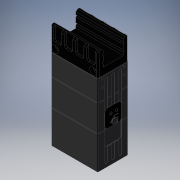
# Autodesk Inventor part: SCHUNK-5521120 Gehaeuse EGP 40
Saved by Autodesk Inventor 2019 (Build 230136000, 136)
## iProperties
Created: 2022-08-29
Part Number: SCHUNK-5521120 Gehaeuse EGP 40
Material: Generic
Catalog Web Link: www.cadenas.de
Description: EGP-Electrical 2-finger parallel gripper
Vendor: SCHUNK
Document SubType Name: Modeling
Designer: psAdmin
Manufacturer: SCHUNK
Mass: 78.9244 g
Surface Area: 169.69 cm^2
Volume: 78.9244 cm^3
Density: 1 g/cm^3
Appearance: PSOLRGB-175-175-175
Category: PARTsolutions
Company: SCHUNK
Title: SCHUNK-5521120 Gehaeuse EGP 40
Author: Cadenas PARTsolutions
Comments: Electrical 2-finger parallel gripper
PSOL_IDENT_0: {$CADENAS_DATA/23d-libs/schunk/greifsysteme/greifmodule/greifmodule_elektrisch/2_finger_parallelgrei
PSOL_IDENT_1: fer/kleinteilegreifer/egp/egp_geh.prj},197 {VTYP=3D},{NB=SCHUNK-5521120 Gehaeuse EGP 40},{LINA=SCHUN
PSOL_IDENT_2: K-5521120 Gehaeuse EGP 40},{NN=EGP},{DATE=27.06.2022 11:10:53},{GEOMDATE=27.06.2022 11:07:50},{VERSI
PSOL_IDENT_3: ON=},{LINEID=10},{WBVAR=},{WBNUMERIC=}  {NB=SCHUNK-5521120 Gehaeuse EGP 40},{LINA=SCHUNK-5521120 Geh
PSOL_IDENT_4: aeuse EGP 40},{KT=DUMMY},{IDNR=5521120},{TYP=EGP 40},{TYP1=2.000},{TYP2=2.000},{TYP3=3.000},{HUB=16.
PSOL_IDENT_5: 000},{HOEHEFIN=100.650},{LGES=40.000},{LIOL=0.000},{WIOL=0.000},{BGES=26.000},{HGES=88.400},{F1=1.00
PSOL_IDENT_6: 0},{HADG=19.750},{HGGE=18.000},{HMGE=22.600},{HDEC=28.000},{F2=0.300},{H1=13.450},{H2=9.450},{H3=6.0
PSOL_IDENT_7: 00},{B1=17.000},{B2=19.700},{T1=0.900},{F3=1.500},{L1=32.000},{H4=3.750},{D2=6.000},{T2=2.900},{D3=4
PSOL_IDENT_8: .000},{T3=6.000},{L2=10.750},{L3=7.000},{L4=2.500},{H5=11.000},{R1=1.500},{T4=1.750},{B3=18.400},{H7=
PSOL_IDENT_9: 10.000},{H8=6.000},{D7=2.500},{T7=2.500},{T8=3.900},{L6=32.000},{D9=6.000},{T9=2.900},{D10=4.000},{T
PSOL_IDENT_10: 10=8.500},{T11=10.500},{L7=34.400},{AL7=0.000},{L8=20.000},{D12=5.000},{T12=14.400},{D13=4.500},{T13=
PSOL_IDENT_11: 2.500},{SW1=2.000},{TSW1=1.100},{L10=61.100},{T14=0.300},{L11=25.000},{L12=14.600},{L13=4.250},{B4=2
PSOL_IDENT_12: .500},{B5=3.500},{D15=12.000},{L15=6.600},{B15=14.200},{B16=7.100},{B17=0.000},{H15=12.800},{R15=2.5
PSOL_IDENT_13: 00},{F4=0.100},{T15=0.600},{H16=15.400},{H17=3.400},{B18=0.650},{D16=4.600},{T16=0.800},{H18=9.900},
PSOL_IDENT_14: {B19=2.000},{B20=3.000},{D17=2.300},{LTYP=34.500},{BTYP=24.300},{TTYP=0.100},{HTYP=9.300},{ETYP=3.00
PSOL_IDENT_15: 0},{G1=3.000},{G1T=4.000},{G1K=6.000},{G1L1=15.250},{G1L2=10.000},{G2L1=0.000},{D18=0.000},{LADG=0.0
PSOL_IDENT_16: 00},{L20=0.010}
NB: SCHUNK-5521120 Gehaeuse EGP 40
NN: EGP
NT: Electrical 2-finger parallel gripper
NBSYN: SCHUNK-$IDNR. Gehaeuse $TYP.
LINA: SCHUNK-5521120 Gehaeuse EGP 40
CATALOG: SCHUNK
IDNR: 5521120
TYP: EGP 40
TYP1: 2
TYP2: 2
TYP3: 3
HUB: 16
HOEHEFIN: 100.65
LGES: 40
LIOL: 0
WIOL: 0
BGES: 26
HGES: 88.4
F1: 1
HADG: 19.75
HGGE: 18
HMGE: 22.6
HDEC: 28
F2: 0.3
H1: 13.45
H2: 9.45
H3: 6
B1: 17
B2: 19.7
T1: 0.9
F3: 1.5
L1: 32
H4: 3.75
D2: 6
T2: 2.9
D3: 4
T3: 6
L2: 10.75
L3: 7
L4: 2.5
H5: 11
R1: 1.5
T4: 1.75
B3: 18.4
H7: 10
H8: 6
D7: 2.5
T7: 2.5
T8: 3.9
L6: 32
D9: 6
T9: 2.9
D10: 4
T10: 8.5
T11: 10.5
L7: 34.4
AL7: 0
L8: 20
D12: 5
T12: 14.4
D13: 4.5
T13: 2.5
SW1: 2
TSW1: 1.1
L10: 61.1
T14: 0.3
L11: 25
L12: 14.6
L13: 4.25
B4: 2.5
B5: 3.5
D15: 12
L15: 6.6
B15: 14.2
B16: 7.1
B17: 0
H15: 12.8
R15: 2.5
F4: 0.1
T15: 0.6
H16: 15.4
H17: 3.4
B18: 0.65
D16: 4.6
T16: 0.8
H18: 9.9
B19: 2
B20: 3
D17: 2.3
LTYP: 34.5
BTYP: 24.3
TTYP: 0.1
HTYP: 9.3
ETYP: 3
G1: 3
G1T: 4
G1K: 6
G1L1: 15.25
G1L2: 10
G2L1: 0
D18: 0
LADG: 0
L20: 0.01
SUPPLIER: SCHUNK
ARTICLENO: SCHUNK-5521120 Gehaeuse EGP 40
BOMINFO: SCHUNK-5521120 Gehaeuse EGP 40
CREATOR: CADENAS GmbH
Autodesk Inventor part; units mm, degrees
sketch "Sketch_1" plane through (0, 0, 0) normal (0, 1, 0) x (-1, 0, 0)
  line L0 (20, -12) -> (20, 12)
  line L1 (20, 12) -> (19, 13)
  line L2 (19, 13) -> (-19, 13)
  line L3 (-19, 13) -> (-20, 12)
  line L4 (-20, 12) -> (-20, -12)
  line L5 (-20, -12) -> (-19, -13)
  line L6 (-19, -13) -> (19, -13)
  line L7 (19, -13) -> (20, -12)
  constraints: 16 end point
extrude "Extrusion1" add sketch "Sketch_1" along normal blind 88.4
sketch "Sketch_25" plane through (0, 88.4, 0) normal (0, 1, 0) x (1, 0, 0)
  circle A0 centre (0, 0) radius 40
  line L0 (-20, 11.9) -> (-20, -11.9)
  line L1 (-20, -11.9) -> (-18.9, -13)
  line L2 (-18.9, -13) -> (18.9, -13)
  line L3 (18.9, -13) -> (20, -11.9)
  line L4 (20, -11.9) -> (20, 11.9)
  line L5 (20, 11.9) -> (18.9, 13)
  line L6 (18.9, 13) -> (-18.9, 13)
  line L7 (-18.9, 13) -> (-20, 11.9)
  constraints: 16 end point, 1 centre point
extrude "Extrusion2" cut sketch "Sketch_25" against normal blind 19.75
sketch "Sketch_3" plane through (0, 0, 0) normal (1, 0, 0) x (0, 1, 0)
  line L0 (88.4, 18) -> (-5, 18)
  line L1 (-5, 18) -> (-5, -18)
  line L2 (-5, -18) -> (88.4, -18)
  line L3 (88.4, -18) -> (88.4, -12.99)
  line L4 (88.4, -12.99) -> (68.89, -12.99)
  line L5 (68.89, -12.99) -> (68.6, -12.7)
  line L6 (68.6, -12.7) -> (68.3, -13)
  line L7 (68.3, -13) -> (50.9, -13)
  line L8 (50.9, -13) -> (50.6, -12.7)
  line L9 (50.6, -12.7) -> (50.3, -13)
  line L10 (50.3, -13) -> (28.3, -13)
  line L11 (28.3, -13) -> (28, -12.7)
  line L12 (28, -12.7) -> (27.7, -13)
  line L13 (27.7, -13) -> (0.3, -13)
  line L14 (0.3, -13) -> (0, -12.7)
  line L15 (0, -12.7) -> (0, 12.7)
  line L16 (0, 12.7) -> (0.3, 13)
  line L17 (0.3, 13) -> (27.7, 13)
  line L18 (27.7, 13) -> (28, 12.7)
  line L19 (28, 12.7) -> (28.3575, 13)
  line L20 (28.3575, 13) -> (50.3, 13)
  line L21 (50.3, 13) -> (50.6, 12.7)
  line L22 (50.6, 12.7) -> (50.9, 13)
  line L23 (50.9, 13) -> (68.3, 13)
  line L24 (68.3, 13) -> (68.6, 12.7)
  line L25 (68.6, 12.7) -> (68.89, 12.99)
  line L26 (68.89, 12.99) -> (88.4, 12.99)
  line L27 (88.4, 12.99) -> (88.4, 18)
  constraints: 56 end point
extrude "Extrusion3" cut sketch "Sketch_3" along normal mid plane 40
sketch "Sketch_4" plane through (0, 0, 0) normal (0, 0, 1) x (1, 0, 0)
  line L0 (-25, 88.4) -> (-25, -5)
  line L1 (-25, -5) -> (25, -5)
  line L2 (25, -5) -> (25, 88.4)
  line L3 (25, 88.4) -> (19.99, 88.4)
  line L4 (19.99, 88.4) -> (19.99, 68.89)
  line L5 (19.99, 68.89) -> (19.7, 68.6)
  line L6 (19.7, 68.6) -> (20, 68.3)
  line L7 (20, 68.3) -> (20, 50.9)
  line L8 (20, 50.9) -> (19.7, 50.6)
  line L9 (19.7, 50.6) -> (20, 50.3)
  line L10 (20, 50.3) -> (20, 28.3)
  line L11 (20, 28.3) -> (19.7, 28)
  line L12 (19.7, 28) -> (20, 27.7)
  line L13 (20, 27.7) -> (20, 0.3)
  line L14 (20, 0.3) -> (19.7, 0)
  line L15 (19.7, 0) -> (-19.7, 0)
  line L16 (-19.7, 0) -> (-20, 0.3)
  line L17 (-20, 0.3) -> (-20, 27.7)
  line L18 (-20, 27.7) -> (-19.7, 28)
  line L19 (-19.7, 28) -> (-20, 28.3575)
  line L20 (-20, 28.3575) -> (-20, 50.3)
  line L21 (-20, 50.3) -> (-19.7, 50.6)
  line L22 (-19.7, 50.6) -> (-20, 50.9)
  line L23 (-20, 50.9) -> (-20, 68.3)
  line L24 (-20, 68.3) -> (-19.7, 68.6)
  line L25 (-19.7, 68.6) -> (-19.99, 68.89)
  line L26 (-19.99, 68.89) -> (-19.99, 88.4)
  line L27 (-19.99, 88.4) -> (-25, 88.4)
  constraints: 56 end point
extrude "Extrusion4" cut sketch "Sketch_4" along normal mid plane 40
sketch "Sketch_2" plane through (0, 0, 0) normal (1, 0, 0) x (0, 1, 0)
  line L0 (86.9, 13) -> (88.4, 11.5)
  line L1 (88.4, 11.5) -> (88.4, 9.85)
  line L2 (88.4, 9.85) -> (87.05, 8.5)
  line L3 (87.05, 8.5) -> (85, 8.5)
  line L4 (85, 8.5) -> (84.1, 9.4)
  line L5 (84.1, 9.4) -> (83.2, 8.5)
  line L6 (83.2, 8.5) -> (79, 8.5)
  line L7 (79, 8.5) -> (78.1, 9.4)
  line L8 (78.1, 9.4) -> (77.2, 8.5)
  line L9 (77.2, 8.5) -> (74.95, 8.5)
  line L10 (74.95, 8.5) -> (74.95, -8.5)
  line L11 (74.95, -8.5) -> (77.2, -8.5)
  line L12 (77.2, -8.5) -> (78.1, -9.4)
  line L13 (78.1, -9.4) -> (79, -8.5)
  line L14 (79, -8.5) -> (83.2, -8.5)
  line L15 (83.2, -8.5) -> (84.1, -9.4)
  line L16 (84.1, -9.4) -> (85, -8.5)
  line L17 (85, -8.5) -> (87.05, -8.5)
  line L18 (87.05, -8.5) -> (88.4, -9.85)
  line L19 (88.4, -9.85) -> (88.4, -11.5)
  line L20 (88.4, -11.5) -> (86.9, -13)
  line L21 (86.9, -13) -> (93.4, -13)
  line L22 (93.4, -13) -> (93.4, 13)
  line L23 (93.4, 13) -> (86.9, 13)
  constraints: 48 end point
extrude "Extrusion5" cut sketch "Sketch_2" along normal mid plane 40
sketch "Sketch_5" plane through (16, 0, 0) normal (1, 0, 0) x (0, 0, -1)
  line L0 (13, 72.4) -> (-13, 72.4)
  line L1 (-13, 72.4) -> (-13, 75.4)
  line L2 (-13, 75.4) -> (-10.1, 75.4)
  line L3 (-10.1, 75.4) -> (-10.1, 74.021)
  line L4 (-10.1, 74.021) -> (13, 74.021)
  line L5 (13, 74.021) -> (13, 72.4)
  line L6 (13, 72.4) -> (-13, 72.4)
  constraints: 14 end point
revolve "Revolution1" cut sketch "Sketch_5" angle 360 about axis through (16, 72.4, -13) along (0, 0, -1)
thread "Thread1" size "M4x0.7" class "6H" standard "ISO Metric profile" length 6
pattern_linear "Rectangular Pattern1" count 2 spacing 32 along (-1, 0, 0) of "Revolution1"
sketch "Sketch_7" plane through (0, 0, 13) normal (0, 0, 1) x (1, 0, 0)
  arc A0 (-17.75, 78.9) -> (-16.25, 77.4) centre (-16.25, 78.9) ccw
  line L0 (-16.25, 77.4) -> (-12.25, 77.4)
  arc A1 (-12.25, 77.4) -> (-10.75, 78.9) centre (-12.25, 78.9) ccw
  line L1 (-10.75, 78.9) -> (-10.75, 88.4)
  line L2 (-10.75, 88.4) -> (-17.75, 88.4)
  line L3 (-17.75, 88.4) -> (-17.75, 78.9)
  constraints: 8 end point, 4 point on circle, 2 centre point
extrude "Extrusion6" cut sketch "Sketch_7" against normal blind 1.75
pattern_linear "Rectangular Pattern2" count 4 spacing 9.5 along (1, 0, 0) of "Extrusion6"
sketch "Sketch_10" plane through (0, 0, -13) normal (0, 0, 1) x (1, 0, 0)
  arc A0 (-17.75, 78.9) -> (-16.25, 77.4) centre (-16.25, 78.9) ccw
  line L0 (-16.25, 77.4) -> (-12.25, 77.4)
  arc A1 (-12.25, 77.4) -> (-10.75, 78.9) centre (-12.25, 78.9) ccw
  line L1 (-10.75, 78.9) -> (-10.75, 88.4)
  line L2 (-10.75, 88.4) -> (-17.75, 88.4)
  line L3 (-17.75, 88.4) -> (-17.75, 78.9)
  constraints: 8 end point, 4 point on circle, 2 centre point
extrude "Extrusion7" cut sketch "Sketch_10" along normal blind 1.75
pattern_linear "Rectangular Pattern3" count 4 spacing 9.5 along (1, 0, 0) of "Extrusion7"
sketch "Sketch9" plane through (20, 50.9, -12) normal (1, 0, 0) x (0, 0, -1)
  point P0 (-21.2, 9.7)
hole "Hole1" at (20, 60.6, 9.2) direction (-1, 0, 0) diameter 2.013 depth 3.9 tip angle 124 thread size "M2.5x0.45" class "6H" standard "ISO Metric profile"
pattern_linear "Rectangular Pattern4" count 2 spacing 18.4 along (0, 0, -1) count 2 spacing 6 along (0, 1, 0) of "Hole1"
sketch "Sketch10" plane through (-20, 50.9, -12) normal (-1, 0, 0) x (0, 0, 1)
  point P0 (21.2, 9.7)
hole "Hole2" at (-20, 60.6, 9.2) direction (1, 0, 0) diameter 2.013 depth 3.9 tip angle 124 thread size "M2.5x0.45" class "6H" standard "ISO Metric profile"
pattern_linear "Rectangular Pattern5" count 2 spacing 18.4 along (0, 0, -1) count 2 spacing 6 along (0, 1, 0) of "Hole2"
sketch "Sketch11" plane through (0, 0, 0) normal (0, -1, 0) x (1, 0, 0)
  point P0 (-16, 0)
hole "Hole3" at (-16, 0, 0) direction (0, 1, 0) diameter 3.242 depth 10.5 tip angle 121 counterbore diameter 6 counterbore depth 2.9 thread size "M4x0.7" class "6H" standard "ISO Metric profile"
pattern_linear "Rectangular Pattern6" count 2 spacing 32 along (1, 0, 0) of "Hole3"
sketch "Sketch_17" plane through (0, 0, -10) normal (0, 0, 1) x (1, 0, 0)
  line L0 (-17.2, 11.9) -> (-17.2, 0)
  line L1 (-17.2, 0) -> (-19.7, 0)
  line L2 (-19.7, 0) -> (-19.7, 14.4)
  line L3 (-19.7, 14.4) -> (-19.45, 14.4)
  line L4 (-19.45, 14.4) -> (-19.45, 12.2)
  arc A0 (-19.45, 12.2) -> (-19.15, 11.9) centre (-19.15, 12.2) ccw
  line L5 (-19.15, 11.9) -> (-17.2, 11.9)
  line L6 (-17.2, 11.9) -> (-17.2, 0)
  constraints: 14 end point, 2 point on circle, 1 centre point
revolve "Revolution2" cut sketch "Sketch_17" angle 360 about axis through (-17.2, 11.9, -10) along (0, 1, 0)
pattern_linear "Rectangular Pattern7" count 2 spacing 34.4 along (1, 0, 0) count 2 spacing 20 along (0, 0, 1) of "Revolution2"
sketch "Sketch_18" plane through (0, 11.9, 0) normal (0, 1, 0) x (1, 0, 0)
  line L0 (-18.2, -10.5774) -> (-17.2, -11.1547)
  line L1 (-17.2, -11.1547) -> (-16.2, -10.5774)
  line L2 (-16.2, -10.5774) -> (-16.2, -9.4226)
  line L3 (-16.2, -9.4226) -> (-17.2, -8.8453)
  line L4 (-17.2, -8.8453) -> (-18.2, -9.4226)
  line L5 (-18.2, -9.4226) -> (-18.2, -10.5774)
  constraints: 12 end point
extrude "Extrusion8" cut sketch "Sketch_18" along normal blind 1.1
pattern_linear "Rectangular Pattern8" count 2 spacing 34.4 along (1, 0, 0) count 2 spacing 20 along (0, 0, -1) of "Extrusion8"
sketch "Sketch_84" plane through (19.7, 0, 0) normal (1, 0, 0) x (0, 0, -1)
  line L0 (-1.25, 65.35) -> (-1.25, 4.25)
  arc A0 (-1.25, 4.25) -> (1.25, 4.25) centre (0, 4.25) ccw
  line L1 (1.25, 4.25) -> (1.25, 65.35)
  arc A1 (1.25, 65.35) -> (-1.25, 65.35) centre (0, 65.35) ccw
  constraints: 4 end point, 4 point on circle, 2 centre point
extrude "Extrusion9" cut sketch "Sketch_84" along normal blind 0.3
sketch "Design_Steckerseite_SKETCH_1" plane through (19.7, 0, 0) normal (1, 0, 0) x (0, 0, -1)
  line L0 (-7.25, 65.35) -> (-7.25, 4.25)
  arc A0 (-7.25, 4.25) -> (-4.75, 4.25) centre (-6, 4.25) ccw
  line L1 (-4.75, 4.25) -> (-4.75, 65.35)
  arc A1 (-4.75, 65.35) -> (-7.25, 65.35) centre (-6, 65.35) ccw
  constraints: 4 end point, 4 point on circle, 2 centre point
sketch "Design_Steckerseite_SKETCH_2" plane through (19.7, 0, 0) normal (1, 0, 0) x (0, 0, -1)
  line L0 (4.75, 65.35) -> (4.75, 4.25)
  arc A0 (4.75, 4.25) -> (7.25, 4.25) centre (6, 4.25) ccw
  line L1 (7.25, 4.25) -> (7.25, 65.35)
  arc A1 (7.25, 65.35) -> (4.75, 65.35) centre (6, 65.35) ccw
  constraints: 4 end point, 4 point on circle, 2 centre point
extrude "Extrusion10" cut sketch "Design_Steckerseite_SKETCH_1" along normal blind 0.3
extrude "Extrusion11" cut sketch "Design_Steckerseite_SKETCH_2" along normal blind 0.3
sketch "Sketch_86" plane through (-19.7, 0, 0) normal (1, 0, 0) x (0, 0, -1)
  line L0 (-1.25, 65.35) -> (-1.25, 4.25)
  arc A0 (-1.25, 4.25) -> (1.25, 4.25) centre (0, 4.25) ccw
  line L1 (1.25, 4.25) -> (1.25, 65.35)
  arc A1 (1.25, 65.35) -> (-1.25, 65.35) centre (0, 65.35) ccw
  constraints: 4 end point, 4 point on circle, 2 centre point
extrude "Extrusion12" cut sketch "Sketch_86" against normal blind 0.3
sketch "Design_SKETCH_1" plane through (-19.7, 0, 0) normal (1, 0, 0) x (0, 0, -1)
  line L0 (-7.25, 65.35) -> (-7.25, 4.25)
  arc A0 (-7.25, 4.25) -> (-4.75, 4.25) centre (-6, 4.25) ccw
  line L1 (-4.75, 4.25) -> (-4.75, 65.35)
  arc A1 (-4.75, 65.35) -> (-7.25, 65.35) centre (-6, 65.35) ccw
  constraints: 4 end point, 4 point on circle, 2 centre point
sketch "Design_SKETCH_2" plane through (-19.7, 0, 0) normal (1, 0, 0) x (0, 0, -1)
  line L0 (4.75, 65.35) -> (4.75, 4.25)
  arc A0 (4.75, 4.25) -> (7.25, 4.25) centre (6, 4.25) ccw
  line L1 (7.25, 4.25) -> (7.25, 65.35)
  arc A1 (7.25, 65.35) -> (4.75, 65.35) centre (6, 65.35) ccw
  constraints: 4 end point, 4 point on circle, 2 centre point
extrude "Extrusion13" cut sketch "Design_SKETCH_1" against normal blind 0.3
extrude "Extrusion14" cut sketch "Design_SKETCH_2" against normal blind 0.3
sketch "Sketch_13" plane through (0, 0, 0) normal (0, 0, 1) x (1, 0, 0)
  line L0 (20, 21.4) -> (19.7, 21.4)
  line L1 (19.7, 21.4) -> (19.7, 27.4)
  line L2 (19.7, 27.4) -> (20, 27.4)
  line L3 (20, 27.4) -> (20, 21.4)
  line L4 (20, 21.4) -> (19.7, 21.4)
  constraints: 10 end point
revolve "Revolution3" cut sketch "Sketch_13" angle 360 about axis through (20, 21.4, 0) along (1, 0, 0)
sketch "Sketch_31" plane through (20, 0, 0) normal (1, 0, 0) x (0, 0, -1)
  line L0 (-7.1, 28) -> (-7.1, 17.7)
  arc A0 (-7.1, 17.7) -> (-4.6, 15.2) centre (-4.6, 17.7) ccw
  line L1 (-4.6, 15.2) -> (4.6, 15.2)
  arc A1 (4.6, 15.2) -> (7.1, 17.7) centre (4.6, 17.7) ccw
  line L2 (7.1, 17.7) -> (7.1, 28)
  line L3 (7.1, 28) -> (-7.1, 28)
  constraints: 8 end point, 4 point on circle, 2 centre point
extrude "Extrusion15" cut sketch "Sketch_31" against normal blind 0.6
sketch "Sketch_32" plane through (0, 0, 0) normal (0, 0, 1) x (1, 0, 0)
  line L0 (19.3, 28) -> (20, 27.3)
  line L1 (20, 27.3) -> (20, 28.7)
  line L2 (20, 28.7) -> (19.3, 28)
  constraints: 6 end point
extrude "Extrusion16" cut sketch "Sketch_32" along normal mid plane 14.2
sketch "Sketch_33" plane through (20, 0, 0) normal (1, 0, 0) x (0, 0, -1)
  line L0 (-7.1, 28) -> (7.1, 28)
  line L1 (7.1, 28) -> (7.1, 40.9)
  arc A0 (7.1, 40.9) -> (4.6, 43.4) centre (4.6, 40.9) ccw
  line L2 (4.6, 43.4) -> (-4.6, 43.4)
  arc A1 (-4.6, 43.4) -> (-7.1, 40.9) centre (-4.6, 40.9) ccw
  line L3 (-7.1, 40.9) -> (-7.1, 28)
  constraints: 8 end point, 4 point on circle, 2 centre point
extrude "Extrusion17" cut sketch "Sketch_33" against normal blind 0.6
sketch "Sketch_39" plane through (20, 0, 0) normal (1, 0, 0) x (0, 0, -1)
  arc A0 (-6.95, 30.7) -> (-4.45, 28.2) centre (-4.45, 30.7) ccw
  line L0 (-4.45, 28.2) -> (4.45, 28.2)
  arc A1 (4.45, 28.2) -> (6.95, 30.7) centre (4.45, 30.7) ccw
  line L1 (6.95, 30.7) -> (6.95, 40.7)
  arc A2 (6.95, 40.7) -> (4.45, 43.2) centre (4.45, 40.7) ccw
  line L2 (4.45, 43.2) -> (-4.45, 43.2)
  arc A3 (-4.45, 43.2) -> (-6.95, 40.7) centre (-4.45, 40.7) ccw
  line L3 (-6.95, 40.7) -> (-6.95, 30.7)
  constraints: 8 end point, 8 point on circle, 4 centre point
extrude "Extrusion18" add sketch "Sketch_39" against normal blind 1.6
sketch "Sketch_35" plane through (20, 0, 0) normal (1, 0, 0) x (0, 0, -1)
  line L0 (-2.85, 31.5) -> (-2.85, 31.3)
  line L1 (-2.85, 31.3) -> (0.55, 31.3)
  line L2 (0.55, 31.3) -> (0.55, 28.6)
  line L3 (0.55, 28.6) -> (3.85, 28.6)
  line L4 (3.85, 28.6) -> (3.85, 29.9)
  line L5 (3.85, 29.9) -> (4.45, 29.9)
  line L6 (4.45, 29.9) -> (4.45, 30.1)
  line L7 (4.45, 30.1) -> (3.65, 30.1)
  line L8 (3.65, 30.1) -> (3.65, 28.8)
  line L9 (3.65, 28.8) -> (0.75, 28.8)
  line L10 (0.75, 28.8) -> (0.75, 31.3)
  line L11 (0.75, 31.3) -> (3.85, 31.3)
  line L12 (3.85, 31.3) -> (3.85, 32.3)
  line L13 (3.85, 32.3) -> (4.45, 32.3)
  line L14 (4.45, 32.3) -> (4.45, 32.5)
  line L15 (4.45, 32.5) -> (3.65, 32.5)
  line L16 (3.65, 32.5) -> (3.65, 31.5)
  line L17 (3.65, 31.5) -> (0.75, 31.5)
  line L18 (0.75, 31.5) -> (0.75, 34.7)
  line L19 (0.75, 34.7) -> (4.45, 34.7)
  line L20 (4.45, 34.7) -> (4.45, 34.9)
  line L21 (4.45, 34.9) -> (0.55, 34.9)
  line L22 (0.55, 34.9) -> (0.55, 31.5)
  line L23 (0.55, 31.5) -> (-2.85, 31.5)
  constraints: 48 end point
extrude "Extrusion19" cut sketch "Sketch_35" against normal blind 0.1
sketch "Sketch26" plane through (20, 0, 0) normal (1, 0, 0) x (0, 0, -1)
  point P0 (-2, 37.9)
hole "Hole4" at (20, 37.9, 2) direction (-1, 0, 0) diameter 2.3 depth 0.2
pattern_linear "Rectangular Pattern9" count 2 spacing 5 along (0, 0, -1) of "Hole4"
sketch "Sketch_38" plane through (20, 0, 0) normal (1, 0, 0) x (0, 0, -1)
  circle A0 centre (0.65, 31.4) radius 2.3
  constraints: 1 centre point
extrude "Extrusion20" add sketch "Sketch_38" along normal blind 0.8
sketch "Sketch_41" plane through (-5, 0, 0) normal (1, 0, 0) x (0, 0, -1)
  line L0 (50, 73.15) -> (-50, 73.15)
  line L1 (6.2612, 73.15) -> (7, 74.3795)
  line L2 (7, 74.3795) -> (13, 74.3795)
  line L3 (13, 74.3795) -> (13, 73.15)
  line L4 (13, 73.15) -> (6.2612, 73.15)
  constraints: 10 end point
revolve "Revolution4" cut sketch "Sketch_41" angle 360 about axis through (-5, 73.15, -50) along (0, 0, -1)
thread "Thread2" size "M3x0.5" class "6H" standard "ISO Metric profile" length 4
pattern_linear "Rectangular Pattern10" count 2 spacing 10 along (1, 0, 0) of "Revolution4"
sketch "Sketch_26" plane through (0, 0, -13) normal (0, 0, 1) x (1, 0, 0)
  arc A0 (-7.5, 43.8) -> (-7.5, 34.5) centre (-7.5, 39.15) ccw
  line L0 (-7.5, 34.5) -> (7.5, 34.5)
  arc A1 (7.5, 34.5) -> (7.5, 43.8) centre (7.5, 39.15) ccw
  line L1 (7.5, 43.8) -> (-7.5, 43.8)
  constraints: 4 end point, 4 point on circle, 2 centre point
extrude "Extrusion21" cut sketch "Sketch_26" along normal blind 0.1
ref_plane "dummy_XY" through (0, 0, 0) normal (0, 1, 0) x (1, 0, 0)
ref_plane "dummy_YZ" through (0, 0, 0) normal (1, 0, 0) x (0, 0, -1)
ref_plane "dummy_ZX" through (0, 0, 0) normal (0, 0, -1) x (0, 1, 0)
ref_plane "fin_1_XY" through (8, 100.65, 0) normal (1, 0, 0) x (0, 0, -1)
ref_plane "fin_1_YZ" through (8, 100.65, 0) normal (0, 0, -1) x (0, 1, 0)
ref_plane "fin_1_ZX" through (8, 100.65, 0) normal (0, 1, 0) x (1, 0, 0)
ref_plane "fin_2_XY" through (-8, 100.65, 0) normal (1, 0, 0) x (0, 0, -1)
ref_plane "fin_2_YZ" through (-8, 100.65, 0) normal (0, 0, -1) x (0, 1, 0)
ref_plane "fin_2_ZX" through (-8, 100.65, 0) normal (0, 1, 0) x (1, 0, 0)
ref_plane "hal_nhs_1_XY" through (20, 66.6, -9.2) normal (1, 0, 0) x (0, 0, -1)
ref_plane "hal_nhs_1_YZ" through (20, 66.6, -9.2) normal (0, 0, -1) x (0, 1, 0)
ref_plane "hal_nhs_1_ZX" through (20, 66.6, -9.2) normal (0, 1, 0) x (1, 0, 0)
ref_plane "hal_nhs_2_XY" through (20, 66.6, 9.2) normal (1, 0, 0) x (0, 0, -1)
ref_plane "hal_nhs_2_YZ" through (20, 66.6, 9.2) normal (0, 0, -1) x (0, 1, 0)
ref_plane "hal_nhs_2_ZX" through (20, 66.6, 9.2) normal (0, 1, 0) x (1, 0, 0)
ref_plane "klh_XY" through (20, 60.6, 0) normal (1, 0, 0) x (0, 0, -1)
ref_plane "klh_YZ" through (20, 60.6, 0) normal (0, 0, -1) x (0, 1, 0)
ref_plane "klh_ZX" through (20, 60.6, 0) normal (0, 1, 0) x (1, 0, 0)
ref_plane "stecker_XY" through (19.7, 21.4, 0) normal (1, 0, 0) x (0, 0, -1)
ref_plane "stecker_YZ" through (19.7, 21.4, 0) normal (0, 0, -1) x (0, 1, 0)
ref_plane "stecker_ZX" through (19.7, 21.4, 0) normal (0, 1, 0) x (1, 0, 0)
ref_plane "typ_XY" through (0, 39.15, -12.9) normal (0, 0, 1) x (1, 0, 0)
ref_plane "typ_YZ" through (0, 39.15, -12.9) normal (1, 0, 0) x (0, 1, 0)
ref_plane "typ_ZX" through (0, 39.15, -12.9) normal (0, 1, 0) x (0, 0, 1)
ref_plane "typ_50_XY" through (4.5, 39.15, -12.9) normal (0, 0, 1) x (1, 0, 0)
ref_plane "typ_50_YZ" through (4.5, 39.15, -12.9) normal (1, 0, 0) x (0, 1, 0)
ref_plane "typ_50_ZX" through (4.5, 39.15, -12.9) normal (0, 1, 0) x (0, 0, 1)
ref_plane "zhu_seitl_1_XY" through (-16, 72.4, 10.1) normal (0, 0, 1) x (1, 0, 0)
ref_plane "zhu_seitl_1_YZ" through (-16, 72.4, 10.1) normal (1, 0, 0) x (0, 1, 0)
ref_plane "zhu_seitl_1_ZX" through (-16, 72.4, 10.1) normal (0, 1, 0) x (0, 0, 1)
ref_plane "zhu_seitl_2_XY" through (16, 72.4, 10.1) normal (0, 0, 1) x (1, 0, 0)
ref_plane "zhu_seitl_2_YZ" through (16, 72.4, 10.1) normal (1, 0, 0) x (0, 1, 0)
ref_plane "zhu_seitl_2_ZX" through (16, 72.4, 10.1) normal (0, 1, 0) x (0, 0, 1)
ref_plane "zhu_unten_1_XY" through (16, 2.9, 0) normal (0, 1, 0) x (1, 0, 0)
ref_plane "zhu_unten_1_YZ" through (16, 2.9, 0) normal (1, 0, 0) x (0, 0, -1)
ref_plane "zhu_unten_1_ZX" through (16, 2.9, 0) normal (0, 0, -1) x (0, 1, 0)
ref_plane "zhu_unten_2_XY" through (-16, 2.9, 0) normal (0, 1, 0) x (1, 0, 0)
ref_plane "zhu_unten_2_YZ" through (-16, 2.9, 0) normal (1, 0, 0) x (0, 0, -1)
ref_plane "zhu_unten_2_ZX" through (-16, 2.9, 0) normal (0, 0, -1) x (0, 1, 0)
body "Solid1"
